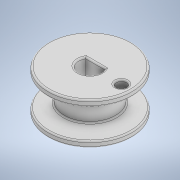
# Autodesk Inventor part: Pulley1
Saved by Autodesk Inventor 2022 (Build 260153000, 153)
## iProperties
Created: 2022-04-05
Part Number: Pulley1
Material: Generic
Document SubType Name: Modeling
Designer: thoms
Density: 1 g/cm^3
Appearance: Default
Author: thoms
Autodesk Inventor part; units mm, degrees
ref_plane "YZ Plane" through (0, 0, 0) normal (1, 0, 0) x (0, 1, 0)
ref_plane "XZ Plane" through (0, 0, 0) normal (0, 1, 0) x (-1, 0, 0)
ref_plane "XY Plane" through (0, 0, 0) normal (0, 0, 1) x (1, 0, 0)
sketch "Sketch1" plane through (0, 0, 0) normal (0, 1, 0) x (-1, 0, 0)
  circle A0 centre (0, 0) radius 4
  dimension "d0" = 8
  constraints: 1 centre point, 1 coincident
  measures "d0" diameter of A0
extrude "Extrusion1" add sketch "Sketch1" along normal blind 4
sketch "Sketch2" plane through (0, 4, 0) normal (0, 1, 0) x (1, 0, 0)
  circle A0 centre (0, 0) radius 1.075
  line L0 (-0.9381, 0.525) -> (0.9381, 0.525)
  dimension "d3" = 2.15
  dimension "d4" = 1.6
  constraints: 2 end point, 2 point on circle, 1 centre point, 1 coincident, 1 horizontal
  measures "d3" diameter of A0
extrude "Extrusion2" cut sketch "Sketch2" against normal up to surface (4 mm away) contours A0 L0 picked at (0.2453, -0.5698)
sketch "Sketch4" plane through (0, 0, 0) normal (0, 0, 1) x (1, 0, 0)
  line L0 (4.4381, 3.5359) -> (2.4381, 3)
  line L1 (2.4381, 3) -> (2.4381, 1)
  line L2 (2.4381, 1) -> (4.4381, 0.4641)
  line L3 (4.4381, 0.4641) -> (4.4381, 3.5359)
  line L4 (0.9381, 4) -> (0.9381, 0) projected
  line L5 (4, 4) -> (-4, 4) projected
  line L6 (4, 0) -> (-4, 0) projected
  line L7 (0, -0.8) -> (0, 4.8) projected
  point P0 (0, 0)
  dimension "d7" = 1.5
  dimension "d8" = 15
  dimension "d9" = 15
  dimension "d10" = 2
  dimension "d11" = 1
  dimension "d12" = 3.5
  constraints: 8 end point, 1 parallel, 1 vertical
  measures "d7" distance between parallel lines of L4 L1
  measures "d8" angle of L5 L0
  measures "d9" angle of L6 L2
  measures "d10" distance of L0.end L1.end
  measures "d11" distance from line of L6 L1.end
  measures "d12" distance between parallel lines of L4 L3
revolve "Revolution1" cut sketch "Sketch4" angle 360 about axis through (0, -10, 0) along (0, 1, 0) contours L3 L2 L1 L0
sketch "Sketch5" plane through (0, 4, 0) normal (0, 1, 0) x (1, 0, 0)
  circle A0 centre (3, 0) radius 0.5
  point P0 (0, 0)
  dimension "d14" = 1
  dimension "d15" = 3
  constraints: 1 centre point
  measures "d14" diameter of A0
  measures "d15" distance of point (0, 0) A0.centre
extrude "Extrusion3" cut sketch "Sketch5" against normal up to surface
fillet "Fillet1" radius 0.15 15 edges at (0, 4, 1.075) (0, 4, -0.525) (4, 4, 0) (0, 3.4185, 4) (0, 3.4185, -4) (0, 0.5815, -4) (0, 0.5815, 4) (4, 0, 0) (-2.4381, 1, 0) (-2.4381, 3, 0) (2.9938, 3.16, -0.5) (2.9939, 3.16, 0.5) (2.5, 4, 0) (0, 0, -0.525) (0, 0, 1.075)
body "Solid1"
